Barrel Nozzle_v4 (Autodesk Fusion 360 design; units mm, degrees)
Autodesk Fusion 360 part; units mm, degrees
note: some values were not read from the file. Set by a fixed rule: which sketch regions a step uses.
sketch "Sketch1" plane through (0, 0, 0) normal (0, 1, 0) x (1, 0, 0)
  circle A0 centre (0, 0) radius 4.7
  circle A1 centre (0, 0) radius 2
  circle A2 centre (15, 0) radius 4.7
  circle A3 centre (15, 0) radius 1.75
  circle A4 centre (0, 15) radius 4.7
  circle A5 centre (0, 15) radius 1.5
  circle A6 centre (15, 15) radius 4.7
  circle A7 centre (15, 15) radius 1.25
  circle A8 centre (0, 0) radius 6.5
  circle A9 centre (15, 0) radius 6.5
  circle A10 centre (0, 15) radius 6.5
  circle A11 centre (15, 15) radius 6.5
  circle A12 centre (-15, 0) radius 6.5
  circle A13 centre (-15, 0) radius 4.7
  circle A14 centre (-15, 15) radius 6.5
  circle A15 centre (-15, 15) radius 4.7
  line L0 (-12, -1) -> (12, -1)
  line L1 (12, -1) -> (12, 1)
  line L2 (12, 1) -> (-12, 1)
  line L3 (-12, 1) -> (-12, -1)
  line L4 (-12, 14) -> (12, 14)
  line L5 (12, 14) -> (12, 16)
  line L6 (12, 16) -> (-12, 16)
  line L7 (-12, 16) -> (-12, 14)
  line L8 (-16, 4) -> (-14, 4)
  line L9 (-14, 4) -> (-14, 11)
  line L10 (-14, 11) -> (-16, 11)
  line L11 (-16, 11) -> (-16, 4)
  line L12 (-1, 4) -> (1, 4)
  line L13 (1, 4) -> (1, 11)
  line L14 (1, 11) -> (-1, 11)
  line L15 (-1, 11) -> (-1, 4)
  line L16 (14, 4) -> (16, 4)
  line L17 (16, 4) -> (16, 11)
  line L18 (16, 11) -> (14, 11)
  line L19 (14, 11) -> (14, 4)
  dimension "d1" = 9.4
  dimension "d2" = 4
  dimension "d3" = 9.4
  dimension "d4" = 3.5
  dimension "d5" = 9.4
  dimension "d6" = 3
  dimension "d7" = 9.4
  dimension "d8" = 2.5
  dimension "d11" = 13
  dimension "d12" = 13
  dimension "d13" = 13
  dimension "d14" = 13
  dimension "d27" = 13
  dimension "d28" = 9.4
  dimension "d31" = 13
  dimension "d32" = 9.4
  constraint coincident A0.centre A1.centre
  constraint concentric A0 A1
  constraint concentric A2 A3
  constraint concentric A4 A5
  constraint concentric A6 A7
  constraint concentric A1 A8
  constraint concentric A2 A9
  constraint concentric A5 A10
  constraint concentric A7 A11
  constraint concentric A12 A13
  constraint concentric A14 A15
  constraint horizontal L0
  constraint vertical L1
  constraint horizontal L2
  constraint vertical L3
  constraint horizontal L4
  constraint vertical L5
  constraint horizontal L6
  constraint vertical L7
  constraint horizontal L8
  constraint vertical L9
  constraint horizontal L10
  constraint vertical L11
  constraint horizontal L12
  constraint vertical L13
  constraint horizontal L14
  constraint vertical L15
  constraint horizontal L16
  constraint vertical L17
  constraint horizontal L18
  constraint vertical L19
  measures "d1" diameter of A0
  measures "d2" diameter of A1
  measures "d3" diameter of A2
  measures "d4" diameter of A3
  measures "d5" diameter of A4
  measures "d6" diameter of A5
  measures "d7" diameter of A6
  measures "d8" diameter of A7
  measures "d11" diameter of A8
  measures "d12" diameter of A9
  measures "d13" diameter of A10
  measures "d14" diameter of A11
  measures "d27" diameter of A12
  measures "d28" diameter of A13
  measures "d31" diameter of A14
  measures "d32" diameter of A15
extrude "Extrude1" add sketch "Sketch1" along normal blind 20 contours A0 A1 L0 L2 | A0 A1 L2 L12 L13 L15 | A0 A1 L0 | A0 L12 L13 L15 | A0 A1 L0 L2 | A2 L0 L1 L2 | A2 L0 L1 L2 L16 L17 L19 | A4 A5 L4 L13 L14 L15 | A4 L13 L14 L15 | A2 L16 L17 L19 | A13 L0 L2 L3 | A13 L0 L2 L3 L8 L9 L11 | A4 A5 L4 L6 | A6 L17 L18 L19 | A6 L4 L5 L6 L17 L18 L19 | A13 L8 L9 L11 | A4 A5 L4 L6 | A6 L4 L5 L6 | A15 L9 L10 L11 | A15 L4 L6 L7 L9 L10 L11 | A4 A5 L6 | A15 L4 L6 L7 makes body 1 at (19.6766, 6.6667, 0.468) makes body 2 at (4.6766, 6.6667, -14.532) makes body 3 at (4.6766, 6.6667, 0.468) makes body 4 at (19.6766, 13.3333, -15.468) makes body 5 at (-10.3234, 6.6667, 0.468) makes body 6 at (-10.3234, 6.6667, -14.532)
extrude "Extrude2" add sketch "Sketch1" against normal blind 10 contours A0 A1 L0 L2 | A0 A8 L0 L2 | A0 A1 L2 L12 L13 L15 | A0 A8 L2 L13 | A0 A8 L0 | A0 A1 L0 | A0 L12 L13 L15 | A0 A8 L13 L15 | A0 A8 L0 L2 | A0 A1 L0 L2 | A0 A8 L2 L15 | A2 A9 L0 L2 | A2 A9 L2 L19 | A2 A9 L0 L17 | A4 A10 L4 L13 | A4 A10 L13 L15 | A2 A9 L17 L19 | A2 L0 L1 L2 | A2 L0 L1 L2 L16 L17 L19 | A12 A13 L0 L2 | A12 A13 L0 L11 | A4 A10 L4 L15 | A4 A10 L4 L6 | A4 A5 L4 L13 L14 L15 | A4 L13 L14 L15 | A6 A11 L17 L19 | A6 A11 L4 L19 | A2 L16 L17 L19 | A12 A13 L2 L9 | A12 A13 L9 L11 | A13 L0 L2 L3 | A13 L0 L2 L3 L8 L9 L11 | A4 A10 L4 L6 | A4 A5 L4 L6 | A6 A11 L4 L6 | A6 A11 L6 L17 | A6 L17 L18 L19 | A6 L4 L5 L6 L17 L18 L19 | A14 A15 L9 L11 | A14 A15 L6 L11 | A13 L8 L9 L11 | A4 A10 L6 | A14 A15 L4 L6 | A14 A15 L4 L9 | A4 A5 L4 L6 | A6 L4 L5 L6 | A15 L9 L10 L11 | A15 L4 L6 L7 L9 L10 L11 | A4 A5 L6 | A15 L4 L6 L7 bodies 4 3 5 2 1 6
chamfer "Chamfer1" distance 2 angle 45 4 edges at (-6.0601, -10, -2.3505) (8.9399, -10, -2.3505) (-6.0601, -10, -17.3505) (8.9399, -10, -17.3505) measured on face at (4.9684, -10, 0.4223) measured on face at (19.8925, -10, 0.3229) measured on face at (4.8091, -10, -14.6771) measured on face at (19.7211, -10, -14.615) on bodies 1 2 3 4 5 6
chamfer "Chamfer1" distance 2 angle 45 1 edges at (-21.0601, -10, -2.3505) measured on face at (-15.0772, -10, -1.5985) on bodies 1 2 3 4 5 6
chamfer "Chamfer1" distance 2 angle 45 1 edges at (-21.0601, -10, -17.3505) measured on face at (-16.9806, -10, -13.1623) on bodies 1 2 3 4 5 6
chamfer "Chamfer2" distance 2.95 angle 45 1 edges at (13.3684, 20, -0.6328) measured on face at (18.6992, 20, -0.2335) on bodies 1
chamfer "Chamfer3" distance 2.7 angle 45 1 edges at (-1.8647, 20, -0.7232) measured on face at (3.7825, 20, -0.2335) on bodies 3
chamfer "Chamfer4" distance 3.45 angle 45 1 edges at (13.8346, 20, -15.452) measured on face at (18.5278, 20, -15.2956) on bodies 4
chamfer "Chamfer5" distance 3.2 angle 45 1 edges at (-1.3985, 20, -15.5424) measured on face at (3.6158, 20, -15.2335) on bodies 2
extrude "Extrude3" add sketch "Sketch1" along normal blind 0.5 from surface at -10 contours A0 A1 L0 L2 | A0 A8 L0 L2 | A0 L12 L13 L15 | A0 A8 L13 L15 | A8 A9 L0 L2 | A0 A8 L0 L2 | A0 A1 L0 L2 | A8 A10 L13 L15 | A2 A9 L0 L2 | A8 A12 L0 L2 | A4 A10 L13 L15 | A9 A11 L17 L19 | A2 A9 L17 L19 | A2 L0 L1 L2 | A12 A13 L0 L2 | A4 A10 L4 L6 | A10 A11 L4 L6 | A4 L13 L14 L15 | A6 A11 L17 L19 | A2 L16 L17 L19 | A12 A14 L9 L11 | A12 A13 L9 L11 | A13 L0 L2 L3 | A10 A14 L4 L6 | A4 A10 L4 L6 | A4 A5 L4 L6 | A6 A11 L4 L6 | A6 L17 L18 L19 | A14 A15 L9 L11 | A13 L8 L9 L11 | A14 A15 L4 L6 | A4 A5 L4 L6 | A6 L4 L5 L6 | A15 L9 L10 L11 | A15 L4 L6 L7 bodies 4 3 5 2 1 6
extrude "Extrude4" add sketch "Sketch1" against normal blind 0.5 contours A0 A8 L0 L2 | A0 A8 L13 L15 | A8 A9 L0 L2 | A0 A8 L0 L2 | A8 A10 L13 L15 | A2 A9 L0 L2 | A8 A12 L0 L2 | A4 A10 L13 L15 | A9 A11 L17 L19 | A2 A9 L17 L19 | A12 A13 L0 L2 | A4 A10 L4 L6 | A10 A11 L4 L6 | A6 A11 L17 L19 | A12 A14 L9 L11 | A12 A13 L9 L11 | A10 A14 L4 L6 | A4 A10 L4 L6 | A6 A11 L4 L6 | A14 A15 L9 L11 | A14 A15 L4 L6 bodies 4
